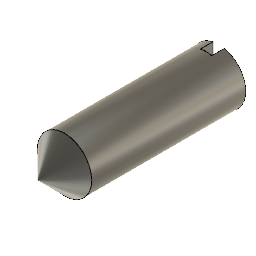
_small.4bb2255b-ea16-4a39-aa88-9f217ea1c4dd (Autodesk Fusion 360 design; units mm, degrees)
Autodesk Fusion 360 part; units mm, degrees
sketch "Sketch1" plane through (0, 0, 0) normal (0, 1, 0) x (1, 0, 0)
  circle A0 centre (0, 0) radius 3
  dimension "d1" = 6
  constraint coincident A0.centre origin
  measures "d1" diameter of A0
extrude "Extrude1" add sketch "Sketch1" along normal blind 20
chamfer "Chamfer1" distance 3 angle 45 1 edges at (-2.797, 0, 1.0848)
ref_plane "WorkPlane1" through (0, 0, 3) normal (0, 0, 1) x (1, 0, 0)
sketch "Sketch2" plane through (0, 0, 3) normal (0, 0, 1) x (1, 0, 0)
  line L0 (3, 20) -> (-3, 20)
  line L1 (0, 20) -> (0, 18.6)
  line L2 (0, 18.6) -> (0.625, 18.6)
  line L3 (0.625, 18.6) -> (0.625, 20)
  line L4 (0.625, 20) -> (-0.605, 20)
  line L5 (-0.605, 20) -> (-0.605, 18.6)
  line L6 (-0.605, 18.6) -> (0.625, 18.6)
  dimension "d6" = 1.4
  dimension "d7" = 0.625
  dimension "d8" = 1.23
  dimension "d9" = 1.4
  constraint midpoint L0 L1.start
  constraint perpendicular L0 L1
  constraint perpendicular L1 L2
  constraint coincident L0 L3.end
  constraint perpendicular L0 L3
  constraint perpendicular L1 L4
  constraint perpendicular L4 L5
  measures "d6" distance of L1.start L1.end
  measures "d7" distance of L1.end L2.end
  measures "d8" distance of L3.end L4.end
  measures "d9" distance of L4.end L5.end
extrude "Extrude2" cut sketch "Sketch2" against normal blind 7
